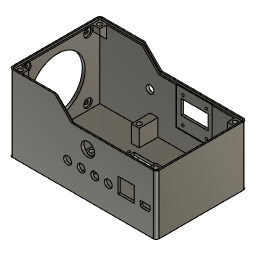
enclosure_bottom (Autodesk Fusion 360 design; units mm, degrees)
Autodesk Fusion 360 part; units mm, degrees
note: some values were not read from the file. Chosen so that the rebuilt part matches the saved one: which face or edge a step refers to. Set by a fixed rule: which sketch regions a step uses.
sketch "Skizze1" plane through (0, 0, 0) normal (0, 0, 1) x (1, 0, 0)
  line L0 (0, 0) -> (130, 0)
  line L1 (130, 0) -> (130, 80)
  line L2 (130, 80) -> (0, 80)
  line L3 (0, 80) -> (0, 0)
  dimension "d1" = 80
  dimension "d2" = 130
  constraint horizontal L0
  constraint vertical L1
  constraint horizontal L2
  constraint vertical L3
  constraint coincident L0.start L3.end
  measures "d1" distance of L0.start L2.end
  measures "d2" distance of L0.start L0.end
  measures "d50" distance of L0.start
extrude "Extrusion1" add sketch "Skizze1" along normal blind 67.5 makes body 1
sketch "Skizze2" plane through (0, 0, 0) normal (0, -1, 0) x (1, 0, 0)
  line L0 (0, 0) -> (130, 0)
  line L1 (130, 0) -> (130, 67.5)
  line L2 (130, 67.5) -> (0, 67.5)
  line L3 (0, 67.5) -> (0, 0)
  line L4 (130, 67.5) -> (40, 67.5)
  line L5 (40, 67.5) -> (55, 52.5)
  line L6 (40, 67.5) -> (70.3522, 67.5) construction
  line L7 (55, 52.5) -> (130, 52.5)
  line L8 (130, 67.5) -> (130, 52.5)
  dimension "d5" = 45
  dimension "d6" = 40
  dimension "d7" = 15
  constraint coincident L1.end L2.start
  constraint coincident L2 L4.end
  constraint perpendicular L1 L4
  constraint horizontal L6
  constraint coincident L1 L7.end
  constraint perpendicular L1 L7
  measures "d5" angle of L5 L6
  measures "d6" distance of L2.end L4.end
  measures "d7" distance of L7.end L1.end
extrude "Extrusion2" cut sketch "Skizze2" against normal blind 90 contours L1 L2 L4 L5 L7 L8 bodies 1
shell "Schale1" thickness 2.5 removed faces 3 at (45, 26.6667, 62.5) at (13.3333, 53.3333, 67.5) at (80, 53.3333, 52.5) on bodies 1
sketch "Skizze3" plane through (0, 0, 52.5) normal (0, 0, 1) x (-1, 0, 0)
  line L0 (-127.5, -77.5) -> (-127.5, -2.5)
  line L1 (-127.5, -2.5) -> (-55, -2.5)
  line L2 (-55, -2.5) -> (-55, 0)
  line L3 (-55, 0) -> (-130, 0)
  line L4 (-130, 0) -> (-130, -80)
  line L5 (-55, -78.8) -> (-127.5, -78.8)
  line L6 (-128.8, -77.5) -> (-128.8, -2.5)
  line L7 (-127.5, -1.2) -> (-55, -1.2)
  line L8 (-55, -1.2) -> (-55, -78.8)
  arc A0 (-128.8, -77.5) -> (-127.5, -78.8) centre (-127.5, -77.5) ccw
  arc A1 (-127.5, -1.2) -> (-128.8, -2.5) centre (-127.5, -2.5) ccw
  line L9 (-55, -77.5) -> (-127.5, -77.5)
  line L10 (-130, -80) -> (-55, -80)
  line L11 (-55, -80) -> (-55, -77.5)
  point P0 (-127.5, -2.5)
  point P1 (-127.5, -77.5)
  point P2 (-127.5, -2.5)
  point P3 (-127.5, -77.5)
  dimension "d13" = 1.2
  constraint horizontal L5
  constraint vertical L6
  constraint horizontal L7
  constraint vertical L8
  constraint tangent L5 A0
  constraint tangent L6 A0
  constraint tangent L7 A1
  constraint tangent L6 A1
  constraint equal A0 A1
  constraint coincident P3 L0.start
  measures "d13" distance of L2.end L7.end
extrude "Extrusion3" cut sketch "Skizze3" against normal blind 1.7 contours L0 L1 L2 L5 L6 L7 L8 A0 A1 L9 L11 bodies 1
sketch "Skizze4" plane through (0, 0, 67.5) normal (0, 0, 1) x (-1, 0, 0)
  line L0 (-40, -77.5) -> (-40, -80)
  line L1 (-40, -80) -> (0, -80)
  line L2 (0, -80) -> (0, 0)
  line L3 (0, 0) -> (-40, 0)
  line L4 (-40, 0) -> (-40, -2.5)
  line L5 (-40, -2.5) -> (-2.5, -2.5)
  line L6 (-40, -78.8) -> (-40, -1.2)
  line L7 (-40, -78.8) -> (-2.5, -78.8)
  line L8 (-1.2, -77.5) -> (-1.2, -2.5)
  line L9 (-2.5, -1.2) -> (-40, -1.2)
  arc A0 (-2.5, -78.8) -> (-1.2, -77.5) centre (-2.5, -77.5) ccw
  arc A1 (-1.2, -2.5) -> (-2.5, -1.2) centre (-2.5, -2.5) ccw
  point P0 (-2.5, -77.5)
  dimension "d18" = 1.2
  dimension "d158" = 1.2
  constraint vertical L6
  constraint coincident L0 L6.start
  constraint perpendicular L6 L7
  constraint perpendicular L5 L8
  constraint horizontal L9
  constraint tangent L7 A0
  constraint tangent L8 A0
  constraint tangent L8 A1
  constraint tangent L9 A1
  constraint equal A0 A1
  constraint coincident P0 A0.centre
  measures "d18" distance of L3.end L6.end
  measures "d158" distance of L1.end L8
extrude "Extrusion4" cut sketch "Skizze4" against normal blind 1.7 contours L0 L4 L6 L7 L8 L9 A0 A1 bodies 1
sketch "Skizze5" plane through (0, 77.5, 0) normal (0, -1, 0) x (1, 0, 0)
  line L0 (2.5, 65.8) -> (2.5, 2.5)
  line L1 (2.5, 2.5) -> (127.5, 2.5)
  line L2 (127.5, 2.5) -> (127.5, 50.8)
  line L3 (40, 67.5) -> (55, 52.5)
  line L4 (55, 52.5) -> (55, 50.8)
  line L5 (55, 50.8) -> (40, 65.8)
  line L6 (40, 65.8) -> (40, 67.5)
  line L7 (55, 52.5) -> (40, 67.5)
  line L8 (40, 65.8) -> (2.5, 65.8)
  line L9 (127.5, 50.8) -> (55, 50.8)
  line L10 (55, 50.8) -> (55, 52.5)
  line L11 (40, 67.5) -> (40, 65.8)
extrude "Extrusion5" cut sketch "Skizze5" against normal blind 1.3 contours L3 L4 L5 L6 L7 L10 L11 bodies 1
sketch "Skizze6" plane through (0, 2.5, 0) normal (0, 1, 0) x (-1, 0, 0)
  line L0 (-40, 67.5) -> (-55, 52.5)
  line L1 (-55, 52.5) -> (-55, 50.8)
  line L2 (-55, 50.8) -> (-127.5, 50.8)
  line L3 (-127.5, 50.8) -> (-127.5, 2.5)
  line L4 (-127.5, 2.5) -> (-2.5, 2.5)
  line L5 (-2.5, 2.5) -> (-2.5, 65.8)
  line L6 (-2.5, 65.8) -> (-40, 65.8)
  line L7 (-40, 67.5) -> (-55, 52.5)
  line L8 (-55, 52.5) -> (-55, 50.8)
  line L9 (-55, 50.8) -> (-40, 65.8)
  line L10 (-40, 65.8) -> (-40, 67.5)
  line L11 (-40, 65.8) -> (-40, 67.5)
  constraint coincident L0.start L7.start
  constraint coincident L0.end L1.start
  constraint coincident L1.end L2.start
  constraint coincident L6.end L9.end
extrude "Extrusion6" cut sketch "Skizze6" against normal blind 1.3 contours L0 L1 L7 L8 L9 L10 L11 bodies 1
sketch "Skizze7" plane through (0, 0, 0) normal (-1, 0, 0) x (0, -1, 0)
  line L0 (0, 67.5) -> (-80, 67.5)
  line L1 (-80, 35) -> (0, 35) construction
  circle A0 centre (-67, 62) radius 1.6
  circle A1 centre (-13, 62) radius 1.6
  circle A2 centre (-67, 8) radius 1.6
  circle A3 centre (-13, 8) radius 1.6
  circle A4 centre (-40, 35) radius 24.5
  line L2 (-80, 0) -> (0, 0)
  line L3 (-80, 67.5) -> (-80, 0)
  line L4 (0, 0) -> (0, 67.5)
  point P0 (0, 67.5)
  dimension "d27" = 27
  dimension "d30" = 3.2
  dimension "d31" = 49
  dimension "d154" = 27
  dimension "d155" = 27
  dimension "d177" = 32.5
  constraint equal A0 A1
  constraint equal A1 A3
  constraint equal A0 A2
  constraint symmetric L1 A1.centre A3.centre
  constraint symmetric L1 A0.centre A2.centre
  constraint horizontal A0.centre A1.centre
  constraint midpoint L1 A4.centre
  constraint coincident L1.start L3
  constraint coincident L1.end L4
  measures "d27" distance of L1 A1.centre
  measures "d30" diameter of A0
  measures "d31" diameter of A4
  measures "d154" horizontal distance of A1.centre A4.centre
  measures "d155" horizontal distance of A0.centre A4.centre
  measures "d177" distance of L0 L1.end
extrude "Extrusion7" cut sketch "Skizze7" against normal blind 2.5 contours A0 | A1 | A2 | A3 | A4 bodies 1
sketch "Skizze9" plane through (0, 0, 2.5) normal (0, 0, 1) x (-1, 0, 0)
  line L0 (-2.5, -77.5) -> (-2.5, -2.5)
  line L1 (-2.5, -2.5) -> (-127.5, -2.5)
  line L2 (-127.5, -2.5) -> (-127.5, -77.5)
  line L3 (-127.5, -77.5) -> (-2.5, -77.5)
  line L4 (-47, -77.5) -> (-54, -77.5)
  line L5 (-54, -77.5) -> (-54, -61)
  line L6 (-54, -61) -> (-47, -61)
  line L7 (-47, -61) -> (-47, -77.5)
  line L8 (-47, -2.5) -> (-54, -2.5)
  line L9 (-54, -2.5) -> (-54, -26)
  line L10 (-54, -26) -> (-47, -26)
  line L11 (-47, -26) -> (-47, -2.5)
  line L12 (-127.5, -68) -> (-117, -68)
  line L13 (-117, -68) -> (-117, -61)
  line L14 (-117, -61) -> (-127.5, -61)
  line L15 (-127.5, -61) -> (-127.5, -68)
  line L16 (-127.5, -26) -> (-117, -26)
  line L17 (-117, -26) -> (-117, -19)
  line L18 (-117, -19) -> (-127.5, -19)
  line L19 (-127.5, -19) -> (-127.5, -26)
  dimension "d37" = 7
  dimension "d38" = 10.5
  dimension "d39" = 58.5
  dimension "d40" = 16.5
  dimension "d41" = 73.5
  constraint horizontal L4
  constraint vertical L5
  constraint horizontal L6
  constraint vertical L7
  constraint coincident L3 L4.start
  constraint horizontal L8
  constraint vertical L9
  constraint horizontal L10
  constraint vertical L11
  constraint coincident L1 L8.start
  constraint horizontal L12
  constraint vertical L13
  constraint horizontal L14
  constraint vertical L15
  constraint coincident L2 L12.start
  constraint horizontal L16
  constraint vertical L17
  constraint horizontal L18
  constraint vertical L19
  constraint coincident L2 L16.start
  constraint equal L6 L13
  constraint equal L6 L10
  constraint equal L6 L17
  constraint coincident L13.end L17
  constraint coincident L9.end L16
  constraint coincident L5.end L14
  constraint vertical L6.end L10.end
  measures "d37" distance of L9.end L10.end
  measures "d38" distance of L16.start L16.end
  measures "d39" distance of L1 L13.end
  measures "d40" distance of L1 L17.end
  measures "d41" distance of L2 L5.end
extrude "Extrusion9" add sketch "Skizze9" along normal blind 15 contours L3 L4 L5 L6 L7 | L1 L8 L9 L10 L11 | L2 L12 L13 L14 L15 | L2 L16 L17 L18 L19 bodies 1
sketch "Skizze10" plane through (0, 0, 17.5) normal (0, 0, 1) x (-1, 0, 0)
  line L0 (-47, -26) -> (-47, -2.5)
  line L1 (-47, -2.5) -> (-54, -2.5)
  line L2 (-54, -2.5) -> (-54, -26)
  line L3 (-54, -26) -> (-47, -26)
  line L4 (-47, -2.5) -> (-54, -2.5)
  line L5 (-54, -2.5) -> (-54, -18.5)
  line L6 (-54, -18.5) -> (-47, -18.5)
  line L7 (-47, -18.5) -> (-47, -2.5)
  dimension "d44" = 16
  dimension "d45" = 7
  constraint horizontal L4
  constraint vertical L5
  constraint horizontal L6
  constraint vertical L7
  constraint coincident L0.end L1.start
  measures "d44" distance of L0.end L6.end
  measures "d45" distance of L0.end L1.end
extrude "Extrusion10" cut sketch "Skizze10" against normal blind 7.3 contours L0 L1 L2 L4 L5 L6 L7 bodies 1
sketch "Skizze11" plane through (0, 0, 17.5) normal (0, 0, 1) x (-1, 0, 0)
  line L0 (-47, -61) -> (-54, -61)
  line L1 (-54, -61) -> (-54, -77.5)
  line L2 (-54, -77.5) -> (-47, -77.5)
  line L3 (-47, -77.5) -> (-47, -61)
  circle A0 centre (-50.5, -64.5) radius 2
  circle A1 centre (-120.5, -64.5) radius 2
  circle A2 centre (-120.5, -22.5) radius 2
  circle A3 centre (-50.5, -22.5) radius 2
  line L4 (-127.5, -68) -> (-117, -68)
  line L5 (-117, -19) -> (-127.5, -19)
  line L6 (-117, -68) -> (-117, -61)
  dimension "d48" = 3.5
  dimension "d49" = 3.5
  dimension "d50" = 3.5
  dimension "d51" = 3.5
  dimension "d52" = 4
  constraint equal A0 A3
  constraint equal A2 A3
  constraint equal A0 A1
  constraint vertical A0.centre A3.centre
  constraint horizontal A2.centre A3.centre
  constraint vertical A1.centre A2.centre
  constraint horizontal A0.centre A1.centre
  measures "d48" distance of L1 A0.centre
  measures "d49" distance of A1.centre L4
  measures "d50" distance of A2.centre L5
  measures "d51" distance of A1.centre L6
  measures "d52" diameter of A1
extrude "Extrusion11" cut sketch "Skizze11" against normal blind 5 contours A0 | A1 | A2 | A3 bodies 1
sketch "Skizze12" plane through (0, 2.5, 0) normal (0, 1, 0) x (-1, 0, 0)
  line L0 (-47, 10.2) -> (-47, 2.5)
  line L1 (-47, 2.5) -> (-2.5, 2.5)
  line L2 (-2.5, 2.5) -> (-2.5, 65.8)
  line L3 (-2.5, 65.8) -> (-40, 65.8)
  line L4 (-40, 65.8) -> (-55, 50.8)
  line L5 (-55, 50.8) -> (-127.5, 50.8)
  line L6 (-127.5, 50.8) -> (-127.5, 2.5)
  line L7 (-127.5, 2.5) -> (-54, 2.5)
  line L8 (-54, 2.5) -> (-54, 10.2)
  line L9 (-54, 10.2) -> (-47, 10.2)
  line L10 (-127.5, 34.2) -> (-43, 34.2)
  line L11 (-43, 34.2) -> (-43, 10.2)
  line L12 (-43, 10.2) -> (-127.5, 10.2)
  line L13 (-127.5, 10.2) -> (-127.5, 34.2)
  dimension "d55" = 24
  dimension "d152" = 84.5
  constraint horizontal L10
  constraint vertical L11
  constraint horizontal L12
  constraint vertical L13
  constraint coincident L6 L10.start
  constraint coincident L0.start L12
  measures "d55" distance of L10.end L11.end
  measures "d152" distance of L10.start L10.end
extrude "Extrusion12" cut sketch "Skizze12" against normal blind 0.5 contours L6 L9 L10 L11 L12 L13 bodies 1
sketch "Skizze13" plane through (0, 0, 0) normal (0, -1, 0) x (1, 0, 0)
  line L0 (130, 52.5) -> (55, 52.5)
  line L1 (55, 52.5) -> (40, 67.5)
  line L2 (40, 67.5) -> (0, 67.5)
  line L3 (0, 22.2) -> (130, 22.2) construction
  circle A0 centre (51.5, 22.2) radius 3.5
  circle A1 centre (63.5, 22.2) radius 3.5
  circle A2 centre (75.5, 22.2) radius 3.5
  circle A3 centre (87.5, 22.2) radius 3.5
  line L4 (96.1, 18.7) -> (110.5, 18.7)
  line L5 (110.5, 18.7) -> (110.5, 32.4)
  line L6 (110.5, 32.4) -> (96.1, 32.4)
  line L7 (96.1, 32.4) -> (96.1, 18.7)
  line L8 (115.8, 23.7) -> (124.5, 23.7)
  line L9 (124.5, 20.15) -> (123.35, 18.7)
  line L10 (123.35, 18.7) -> (116.95, 18.7)
  line L11 (116.95, 18.7) -> (115.8, 20.15)
  line L12 (115.8, 20.15) -> (115.8, 23.7)
  line L13 (124.5, 23.7) -> (124.5, 20.15)
  circle A4 centre (69.5, 39.6) radius 6.05
  line L14 (0, 67.5) -> (0, 0)
  line L15 (130, 0) -> (0, 0)
  line L16 (130, 0) -> (130, 52.5)
  dimension "d59" = 12
  dimension "d60" = 12
  dimension "d61" = 12
  dimension "d63" = 7
  dimension "d64" = 14.4
  dimension "d65" = 3.5
  dimension "d66" = 10.2
  dimension "d68" = 8.7
  dimension "d69" = 1.15
  dimension "d70" = 1.45
  dimension "d71" = 3.5
  dimension "d73" = 1.5
  dimension "d76" = 12.1
  dimension "d77" = 18
  dimension "d78" = 17.4
  dimension "d178" = 22.2
  dimension "d179" = 5.5
  dimension "d180" = 19.5
  dimension "d181" = 42.5
  constraint coincident L3 A0.centre
  constraint coincident L3 A1.centre
  constraint coincident L3 A2.centre
  constraint coincident L3 A3.centre
  constraint equal A0 A1
  constraint equal A1 A2
  constraint equal A2 A3
  constraint horizontal L4
  constraint vertical L5
  constraint horizontal L6
  constraint vertical L7
  constraint parallel L3 L10
  constraint perpendicular L8 L13
  constraint vertical L12
  constraint horizontal L9.start L11.end
  constraint equal L9 L11
  constraint coincident L3.start L14
  constraint horizontal L3
  constraint horizontal L8
  measures "d59" distance of A0.centre A1.centre
  measures "d60" distance of A1.centre A2.centre
  measures "d61" distance of A2.centre A3.centre
  measures "d63" diameter of A0
  measures "d64" distance of L4.start L4.end
  measures "d65" distance of L3 L4.end
  measures "d66" distance of L3 L5.end
  measures "d68" distance of L8.start L8.end
  measures "d69" horizontal distance of L10.end L11.end
  measures "d70" vertical distance of L10.end L11.end
  measures "d71" distance of L3 L9.end
  measures "d73" distance of L3 L8.end
  measures "d76" diameter of A4
  measures "d77" horizontal distance of A3.centre A4.centre
  measures "d78" distance of L3 A4.centre
  measures "d178" distance of L3.end L15
  measures "d179" distance of L8.end L16
  measures "d180" distance of L5.end L16
  measures "d181" distance of A3.centre L16
extrude "Extrusion13" cut sketch "Skizze13" against normal blind 2.5 contours A0 | A1 | A2 | A3 | L4 L5 L6 L7 | L8 L9 L10 L11 L12 L13 | A4 bodies 1
sketch "Skizze14" plane through (0, 77.5, 0) normal (0, -1, 0) x (1, 0, 0)
  line L0 (54, 17.5) -> (54, 2.5)
  line L1 (54, 2.5) -> (127.5, 2.5)
  line L2 (127.5, 2.5) -> (127.5, 50.8)
  line L3 (55, 50.8) -> (40, 65.8)
  line L4 (2.5, 65.8) -> (2.5, 2.5)
  line L5 (2.5, 2.5) -> (47, 2.5)
  line L6 (47, 2.5) -> (47, 17.5)
  line L7 (47, 17.5) -> (54, 17.5)
  line L8 (70, 18) -> (102, 18)
  line L9 (102, 18) -> (102, 51)
  line L10 (102, 51) -> (70, 51)
  line L11 (70, 51) -> (70, 18)
  line L12 (130, 52.5) -> (55, 52.5)
  line L13 (127.5, 50.8) -> (55, 50.8)
  line L14 (40, 65.8) -> (2.5, 65.8)
  dimension "d79" = 32
  dimension "d81" = 25.5
  dimension "d82" = 33
  dimension "d106" = 1.5
  constraint horizontal L8
  constraint vertical L9
  constraint horizontal L10
  constraint vertical L11
  measures "d79" distance of L8.start L8.end
  measures "d81" distance of L2 L9.end
  measures "d82" distance of L8.end L9.end
  measures "d106" distance of L9.end L12
extrude "Extrusion14" cut sketch "Skizze14" against normal blind 0.5 contours L9 L10 L11 L13 | L8 L9 L11 L13 bodies 1
sketch "Skizze15" plane through (0, 78, 0) normal (0, -1, 0) x (1, 0, 0)
  line L0 (70, 50.8) -> (70, 18)
  line L1 (70, 18) -> (102, 18)
  line L2 (102, 18) -> (102, 50.8)
  line L3 (74, 42) -> (98, 42)
  line L4 (98, 42) -> (98, 29)
  line L5 (98, 29) -> (74, 29)
  line L6 (74, 29) -> (74, 42)
  line L7 (102, 18) -> (70, 18)
  circle A0 centre (75.65, 45.3) radius 1.1
  circle A1 centre (96.35, 45.3) radius 1.1
  circle A2 centre (96.35, 22.1) radius 1.1
  circle A3 centre (75.65, 22.1) radius 1.1
  line L8 (102, 50.8) -> (70, 50.8)
  dimension "d85" = 4
  dimension "d86" = 4
  dimension "d87" = 11
  dimension "d88" = 13
  dimension "d89" = 20.7
  dimension "d90" = 1.65
  dimension "d92" = 3.3
  dimension "d93" = 6.9
  dimension "d94" = 2.2
  constraint horizontal L3
  constraint vertical L4
  constraint horizontal L5
  constraint vertical L6
  constraint equal A0 A1
  constraint equal A1 A2
  constraint equal A2 A3
  constraint horizontal A0.centre A1.centre
  constraint vertical A1.centre A2.centre
  constraint horizontal A2.centre A3.centre
  constraint vertical A0.centre A3.centre
  measures "d85" distance of L0 L3.start
  measures "d86" distance of L2 L4.end
  measures "d87" distance of L4.end L7
  measures "d88" distance of L3.end L4.end
  measures "d89" distance of A0.centre A1.centre
  measures "d90" horizontal distance of L3.end A1.centre
  measures "d92" distance of L3 A1.centre
  measures "d93" distance of L5 A2.centre
  measures "d94" diameter of A1
extrude "Extrusion15" cut sketch "Skizze15" against normal blind 2 contours L3 L4 L5 L6 | A0 | A1 | A2 | A3 bodies 1
sketch "Skizze16" plane through (0, 77.5, 0) normal (0, -1, 0) x (1, 0, 0)
  line L0 (102, 18) -> (70, 18)
  line L1 (70, 18) -> (70, 50.8)
  line L2 (102, 50.8) -> (102, 18)
  line L3 (54, 17.5) -> (54, 2.5)
  line L4 (54, 2.5) -> (127.5, 2.5)
  line L5 (127.5, 2.5) -> (127.5, 50.8)
  line L6 (55, 50.8) -> (40, 65.8)
  line L7 (2.5, 65.8) -> (2.5, 2.5)
  line L8 (2.5, 2.5) -> (47, 2.5)
  line L9 (47, 2.5) -> (47, 17.5)
  line L10 (47, 17.5) -> (54, 17.5)
  circle A0 centre (47, 35.5) radius 3.55
  line L11 (40, 28.5) -> (54, 28.5) construction
  line L12 (54, 28.5) -> (54, 42.5) construction
  line L13 (54, 42.5) -> (40, 42.5) construction
  line L14 (40, 42.5) -> (40, 28.5) construction
  line L15 (70, 50.8) -> (55, 50.8)
  line L16 (40, 65.8) -> (2.5, 65.8)
  line L17 (127.5, 50.8) -> (102, 50.8)
  point P0 (74, 42)
  dimension "d97" = 7.1
  dimension "d98" = 7
  dimension "d99" = 7
  dimension "d100" = 7
  dimension "d101" = 7
  dimension "d107" = 6.5
  constraint horizontal L11
  constraint vertical L12
  constraint horizontal L13
  constraint vertical L14
  constraint vertical L6.end L13.end
  measures "d97" diameter of A0
  measures "d98" distance of A0.centre L12
  measures "d99" distance of A0.centre L14
  measures "d100" distance of A0.centre L13
  measures "d101" distance of A0.centre L11
  measures "d107" vertical distance of A0.centre P0
extrude "Extrusion16" cut sketch "Skizze16" against normal blind 2.5 contours A0 bodies 1
sketch "Skizze17" plane through (0, 0, 2.5) normal (0, 0, 1) x (-1, 0, 0)
  line L0 (-117, -68) -> (-127.5, -68)
  line L1 (-127.5, -68) -> (-127.5, -77.5)
  line L2 (-127.5, -77.5) -> (-54, -77.5)
  line L3 (-54, -77.5) -> (-54, -61)
  line L4 (-54, -61) -> (-47, -61)
  line L5 (-47, -61) -> (-47, -77.5)
  line L6 (-47, -77.5) -> (-2.5, -77.5)
  line L7 (-2.5, -77.5) -> (-2.5, -2.5)
  line L8 (-2.5, -2.5) -> (-47, -2.5)
  line L9 (-47, -2.5) -> (-47, -26)
  line L10 (-47, -26) -> (-54, -26)
  line L11 (-54, -26) -> (-54, -2.5)
  line L12 (-54, -2.5) -> (-127.5, -2.5)
  line L13 (-127.5, -2.5) -> (-127.5, -19)
  line L14 (-127.5, -19) -> (-117, -19)
  line L15 (-117, -19) -> (-117, -26)
  line L16 (-117, -26) -> (-127.5, -26)
  line L17 (-127.5, -26) -> (-127.5, -61)
  line L18 (-127.5, -61) -> (-117, -61)
  line L19 (-117, -61) -> (-117, -68)
  line L20 (-55, -55.5) -> (-121, -55.5)
  line L21 (-121, -55.5) -> (-121, -51.5)
  line L22 (-121, -51.5) -> (-55, -51.5)
  line L23 (-55, -51.5) -> (-55, -55.5)
  circle A0 centre (-52.5, -53.5) radius 1.1
  circle A1 centre (-123.5, -53.5) radius 1.1
  line L24 (0, -40) -> (-130, -40) construction
  line L25 (0, -80) -> (0, 0)
  line L26 (-130, -80) -> (-130, 0)
  circle A2 centre (-15, -40) radius 1.6
  circle A3 centre (-35, -40) radius 1.6
  circle A4 centre (-55, -40) radius 1.6
  circle A5 centre (-75, -40) radius 1.6
  circle A6 centre (-95, -40) radius 1.6
  circle A7 centre (-115, -40) radius 1.6
  circle A8 centre (-117.4, -32) radius 1.6
  circle A9 centre (-15, -32) radius 1.6
  dimension "d108" = 4
  dimension "d109" = 2
  dimension "d110" = 2.5
  dimension "d111" = 2.5
  dimension "d112" = 4
  dimension "d113" = 66
  dimension "d114" = 2.2
  dimension "d115" = 49
  dimension "d116" = 20
  dimension "d117" = 20
  dimension "d118" = 20
  dimension "d119" = 20
  dimension "d120" = 20
  dimension "d121" = 15
  dimension "d122" = 3.2
  dimension "d124" = 15
  dimension "d127" = 3.2
  dimension "d151" = 102.4
  dimension "d156" = 8
  constraint horizontal L20
  constraint vertical L21
  constraint horizontal L22
  constraint vertical L23
  constraint horizontal A0.centre A1.centre
  constraint equal A0 A1
  constraint perpendicular L17 L24
  constraint midpoint L24.start L25
  constraint coincident L24.end L26
  constraint coincident L24 A2.centre
  constraint coincident L24 A3.centre
  constraint coincident L24 A4.centre
  constraint coincident L24 A5.centre
  constraint coincident L24 A6.centre
  constraint coincident L24 A7.centre
  constraint equal A2 A3
  constraint equal A3 A4
  constraint equal A4 A5
  constraint equal A5 A6
  constraint equal A6 A7
  constraint horizontal A8.centre A9.centre
  constraint equal A8 A9
  measures "d108" distance of L20.start L22.end
  measures "d109" distance of L20 A0.centre
  measures "d110" distance of L23 A0.centre
  measures "d111" horizontal distance of L20.end A1.centre
  measures "d112" distance of L17 A1.centre
  measures "d113" distance of L21.end L22.end
  measures "d114" diameter of A0
  measures "d115" distance of L12 L21.end
  measures "d116" distance of A2.centre A3.centre
  measures "d117" distance of A3.centre A4.centre
  measures "d118" distance of A4.centre A5.centre
  measures "d119" distance of A5.centre A6.centre
  measures "d120" distance of A6.centre A7.centre
  measures "d121" distance of L24.end A7.centre
  measures "d122" diameter of A2
  measures "d124" distance of L25 A9.centre
  measures "d127" diameter of A9
  measures "d151" distance of A8.centre A9.centre
  measures "d156" vertical distance of A7.centre A8.centre
extrude "Extrusion17" cut sketch "Skizze17" against normal blind 2.5 contours L20 L21 L22 L23 | A0 | A1 | A2 | A3 | A4 | A5 | A6 | A7 | A8 | A9 bodies 1
sketch "Skizze18" plane through (127.5, 0, 0) normal (-1, 0, 0) x (0, -1, 0)
  line L0 (-68, 2.5) -> (-68, 17.5)
  line L1 (-68, 17.5) -> (-61, 17.5)
  line L2 (-61, 17.5) -> (-61, 2.5)
  line L3 (-61, 2.5) -> (-26, 2.5)
  line L4 (-26, 2.5) -> (-26, 17.5)
  line L5 (-26, 17.5) -> (-19, 17.5)
  line L6 (-19, 17.5) -> (-19, 2.5)
  line L7 (-19, 2.5) -> (-2.5, 2.5)
  line L8 (-2.5, 2.5) -> (-2.5, 10.2)
  line L9 (-2.5, 10.2) -> (-2, 10.2)
  line L10 (-2, 10.2) -> (-2, 34.2)
  line L11 (-2, 34.2) -> (-2.5, 34.2)
  line L12 (-2.5, 34.2) -> (-2.5, 50.8)
  line L13 (-2.5, 50.8) -> (-77.5, 50.8)
  line L14 (-77.5, 50.8) -> (-77.5, 2.5)
  line L15 (-77.5, 2.5) -> (-68, 2.5)
  line L16 (-8.5, 50.8) -> (-2.5, 50.8)
  line L17 (-2.5, 39.8) -> (-8.5, 45.8)
  line L18 (-2.5, 39.8) -> (5.7035, 39.8) construction
  line L19 (-8.5, 45.8) -> (-8.5, 50.8)
  line L20 (-77.5, 50.8) -> (-71.5, 50.8)
  line L21 (-71.5, 45.8) -> (-71.5, 50.8)
  line L22 (-71.5, 45.8) -> (-77.5, 39.8)
  line L23 (-71.5, 45.8) -> (-56.2549, 45.8) construction
  line L24 (-77.5, 50.8) -> (-77.5, 39.8)
  dimension "d130" = 135
  dimension "d132" = 5
  dimension "d133" = 6
  dimension "d134" = 135
  constraint coincident L13 L16.start
  constraint coincident L12.end L13.start
  constraint perpendicular L12 L16
  constraint horizontal L18
  constraint coincident L12 L17.start
  constraint vertical L19
  constraint coincident L13.end L14.start
  constraint coincident L13 L20.end
  constraint perpendicular L13 L21
  constraint horizontal L23
  constraint vertical L24
  constraint equal L19 L21
  constraint equal L16 L20
  measures "d130" angle of L17 L18
  measures "d132" distance of L16.start L17.end
  measures "d133" distance of L13.end L20.end
  measures "d134" angle of L22 L23
extrude "Extrusion18" add sketch "Skizze18" along normal blind 6 contours L13 L14 L20 L21 L22 L24 | L12 L13 L16 L17 L19 bodies 1
sketch "Skizze19" plane through (0, 0, 50.8) normal (0, 0, 1) x (-1, 0, 0)
  line L0 (-121.5, -77.5) -> (-121.5, -71.5)
  line L1 (-121.5, -71.5) -> (-127.5, -71.5)
  line L2 (-127.5, -71.5) -> (-127.5, -8.5)
  line L3 (-127.5, -8.5) -> (-121.5, -8.5)
  line L4 (-121.5, -8.5) -> (-121.5, -2.5)
  line L5 (-121.5, -2.5) -> (-55, -2.5)
  line L6 (-55, -2.5) -> (-55, -1.2)
  line L7 (-55, -1.2) -> (-127.5, -1.2)
  arc A0 (-127.5, -1.2) -> (-128.8, -2.5) centre (-127.5, -2.5) ccw
  line L8 (-128.8, -2.5) -> (-128.8, -77.5)
  arc A1 (-128.8, -77.5) -> (-127.5, -78.8) centre (-127.5, -77.5) ccw
  circle A2 centre (-125, -75) radius 2
  circle A3 centre (-125, -5) radius 2
  line L9 (-130, 0) -> (-55, 0)
  line L10 (-70, -77.5) -> (-70, -78)
  line L11 (-70, -78) -> (-102, -78)
  line L12 (-102, -78) -> (-102, -77.5)
  line L13 (-102, -77.5) -> (-121.5, -77.5)
  line L14 (-127.5, -78.8) -> (-55, -78.8)
  line L15 (-55, -78.8) -> (-55, -77.5)
  line L16 (-55, -77.5) -> (-70, -77.5)
  dimension "d139" = 3.5
  dimension "d140" = 4
  dimension "d160" = 3.5
  dimension "d162" = 3.5
  constraint equal A2 A3
  constraint vertical A2.centre A3.centre
  measures "d139" distance of L3 A3.centre
  measures "d140" diameter of A2
  measures "d160" distance of L0 A2.centre
  measures "d162" distance of L1 A2.centre
extrude "Extrusion19" cut sketch "Skizze19" against normal blind 5 contours A2 | A3 bodies 1
sketch "Skizze21" plane through (2.5, 0, 0) normal (1, 0, 0) x (0, 1, 0)
  circle A0 centre (40, 35) radius 24.5
  circle A1 centre (13, 62) radius 1.6
  circle A2 centre (67, 8) radius 1.6
  circle A3 centre (67, 62) radius 1.6
  circle A4 centre (13, 8) radius 1.6
  line L0 (2.5, 65.8) -> (2.5, 2.5)
  line L1 (2.5, 2.5) -> (77.5, 2.5)
  line L2 (77.5, 2.5) -> (77.5, 65.8)
  circle A5 centre (13, 62) radius 3.8
  circle A6 centre (67, 62) radius 3.8
  circle A7 centre (67, 8) radius 3.8
  circle A8 centre (13, 8) radius 3.8
  line L3 (77.5, 65.8) -> (2.5, 65.8)
  constraint concentric A1 A5
  constraint concentric A3 A6
  constraint concentric A2 A7
  constraint concentric A4 A8
  constraint equal A5 A6
  constraint equal A6 A7
  constraint equal A7 A8
  constraint tangent A5 L3
extrude "Extrusion21" cut sketch "Skizze21" against normal blind 1.3 contours A6 | A5 | A7 | A8 bodies 1
sketch "Skizze22" plane through (2.5, 0, 0) normal (1, 0, 0) x (0, 1, 0)
  line L0 (77.5, 65.8) -> (67, 65.8)
  circle A0 centre (67, 62) radius 3.8
  line L1 (67, 65.8) -> (13, 65.8)
  circle A1 centre (13, 62) radius 3.8
  line L2 (13, 65.8) -> (2.5, 65.8)
  line L3 (2.5, 65.8) -> (2.5, 2.5)
  line L4 (2.5, 2.5) -> (77.5, 2.5)
  line L5 (77.5, 2.5) -> (77.5, 65.8)
  circle A2 centre (40, 35) radius 24.5
  circle A3 centre (13, 8) radius 3.8
  circle A4 centre (67, 8) radius 3.8
  line L6 (77.5, 65.8) -> (71.5, 65.8)
  line L7 (71.5, 65.8) -> (71.5, 60.8)
  line L8 (71.5, 60.8) -> (77.5, 54.8)
  line L9 (71.5, 60.8) -> (79.9853, 60.8) construction
  line L10 (77.5, 54.8) -> (77.5, 65.8)
  line L11 (2.5, 65.8) -> (8.5, 65.8)
  line L12 (8.5, 65.8) -> (8.5, 60.8)
  line L13 (8.5, 60.8) -> (2.5, 54.8)
  line L14 (8.5, 60.8) -> (17.1014, 60.8) construction
  line L15 (2.5, 65.8) -> (2.5, 54.8)
  dimension "d163" = 6
  dimension "d164" = 5
  dimension "d165" = 45
  dimension "d168" = 135
  constraint coincident L0.start L5.end
  constraint perpendicular L5 L6
  constraint perpendicular L0 L7
  constraint horizontal L9
  constraint coincident L5 L8.end
  constraint coincident L2.end L3.start
  constraint perpendicular L3 L11
  constraint perpendicular L2 L12
  constraint horizontal L14
  constraint coincident L3 L13.end
  constraint equal L6 L11
  constraint equal L7 L12
  measures "d163" distance of L0.start L6.end
  measures "d164" distance of L6.end L7.end
  measures "d165" angle of L8 L9
  measures "d168" angle of L13 L14
extrude "Extrusion22" add sketch "Skizze22" along normal blind 6 separate body contours L0 L5 L6 L7 L8 L10 | L2 L3 L11 L12 L13 L15 makes body 2 at (4.5, 77.5, 58.4667) makes body 3 at (4.5, 2.5, 62.1333)
sketch "Skizze23" plane through (0, 0, 65.8) normal (0, 0, 1) x (-1, 0, 0)
  line L0 (-2.5, -77.5) -> (-2.5, -71.5)
  line L1 (-2.5, -71.5) -> (-8.5, -71.5)
  line L2 (-8.5, -71.5) -> (-8.5, -77.5)
  line L3 (-8.5, -77.5) -> (-2.5, -77.5)
  circle A0 centre (-5, -75) radius 2
  circle A1 centre (-5, -5) radius 2
  line L4 (-2.5, -8.5) -> (-8.5, -8.5)
  dimension "d173" = 3.5
  dimension "d174" = 3.5
  dimension "d175" = 3.5
  dimension "d176" = 4
  constraint vertical A0.centre A1.centre
  constraint equal A0 A1
  measures "d173" distance of L2 A0.centre
  measures "d174" distance of L1 A0.centre
  measures "d175" distance of A1.centre L4
  measures "d176" diameter of A0
extrude "Extrusion23" cut sketch "Skizze23" against normal blind 5 contours A0 | A1 bodies 2 3
fillet "Abrundung2" radius 2.5 4 edges at (130, 80, 26.25) (0, 80, 33.75) (130, 0, 26.25) (0, 0, 33.75) on bodies 1
combine "Kombinieren2" operation add target body 1 tool bodies 2 3
imported_body "Abgeleitetes Basiselement1" makes body 4
move_body "Verschieben1" bodies 4 to x (1, 0, 0) y (0, 1, 0) z (0, 0, 1) at (0, 0, 51)
delete_body "Körper entfernen1" bodies 4
named bodies: "Körper1 (1)"
